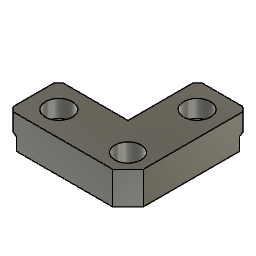
PIU corner bumper v1 (Autodesk Fusion 360 design; units mm, degrees)
Autodesk Fusion 360 part; units mm, degrees
note: some values were not read from the file. Chosen so that the rebuilt part matches the saved one: where a step ends.
sketch "base form" plane through (0, 0, 0) normal (0, 0, 1) x (1, 0, 0)
  line L0 (0, 0) -> (-55, 0)
  line L1 (0, 55) -> (0, 0)
  line L2 (0, 55) -> (-23, 55)
  line L3 (-55, 0) -> (-55, 23)
  line L4 (-55, 23) -> (-23, 23)
  line L5 (-23, 23) -> (-23, 55)
  dimension "d1" = 55
  dimension "d2" = 55
  dimension "d3" = 23
  dimension "d4" = 23
  constraint horizontal L0
  constraint vertical L1
  constraint coincident L0.start L1.end
  constraint perpendicular L1 L2
  constraint perpendicular L0 L3
  constraint horizontal L4
  constraint vertical L5
  measures "d1" distance of L0.start L0.end
  measures "d2" distance of L0.start L1.start
  measures "d3" distance of L1.start L2.end
  measures "d4" distance of L0.end L3.end
extrude "Extrude1" add sketch "base form" along normal blind 15
chamfer "Chamfer1" distance 7 angle 45 1 edges at (0, 0, 7.5)
sketch "frame hole" plane through (0, 0, 15) normal (0, 0, 1) x (-1, 0, 0)
  line L0 (7, 0) -> (0, -7)
  line L1 (0, -7) -> (0, -55)
  line L2 (0, -55) -> (23, -55)
  line L3 (23, -55) -> (23, -23)
  line L4 (23, -23) -> (55, -23)
  line L5 (55, -23) -> (55, 0)
  line L6 (55, 0) -> (7, 0)
  line L7 (3.5, -3.5) -> (5.9749, -5.9749) construction
  line L8 (3.5, -3.5) -> (7, -3.5) construction
  line L9 (5.9749, -5.9749) -> (13.0459, -13.0459) construction
  line L10 (5.9749, -5.9749) -> (15.9749, -5.9749) construction
  circle A0 centre (10.2175, -10.2175) radius 6
  dimension "d8" = 45
  dimension "d9" = 3.5
  dimension "d10" = 45
  dimension "d11" = 10
  dimension "d12" = 12
  constraint horizontal L8
  constraint midpoint L0 L7.start
  constraint horizontal L10
  constraint coincident L7.end A0
  measures "d8" angle of L7 L8
  measures "d9" distance of L7.start L7.end
  measures "d10" angle of L9 L10
  measures "d11" distance of L7.end L9.end
  measures "d12" diameter of A0
sketch "mounting screw holes" plane through (0, 0, 15) normal (0, 0, 1) x (-1, 0, 0)
  line L0 (55, -11.5) -> (49.55, -11.5) construction
  line L1 (55, -23) -> (55, 0) construction
  line L2 (41, 16) -> (41, 11) construction
  line L3 (49.55, -11.5) -> (31, -11.5) construction
  circle A0 centre (43.35, -11.5) radius 6.2
  circle A1 centre (43.35, -11.5) radius 3
  line L4 (3.5, -3.5) -> (10.5711, -10.5711) construction
  line L5 (3.5, -3.5) -> (13.5, -3.5) construction
  line L6 (0, -7) -> (7, 0) construction
  circle A2 centre (11.5, -43.35) radius 6.2
  circle A3 centre (11.5, -43.35) radius 3
  dimension "d13" = 5.45
  dimension "d14" = 5
  dimension "d15" = 12.4
  dimension "d16" = 6
  dimension "d17" = 45
  dimension "d18" = 10
  constraint horizontal L0
  constraint midpoint L0.start L1
  constraint vertical L2
  constraint parallel L0 L3
  constraint coincident L0.end A0
  constraint concentric A0 A1
  constraint horizontal L5
  constraint midpoint L4.start L6
  constraint symmetric A0 L4 A2
  constraint symmetric A1 L4 A3
  measures "d13" distance of L0.start L0.end
  measures "d14" distance of L2.start L2.end
  measures "d15" diameter of A0
  measures "d16" diameter of A1
  measures "d17" angle of L4 L5
  measures "d18" distance of L4.start L4.end
extrude "Extrude2" cut sketch "frame hole" against normal up to surface (15 mm away) contours A0
extrude "Extrude3" cut sketch "mounting screw holes" along normal up to far side of body 1 contours A1 | A3
extrude "Extrude4" cut sketch "mounting screw holes" against normal blind 8
sketch "relief holes" plane through (0, 0, 0) normal (0, 0, -1) x (1, 0, 0)
  circle A0 centre (-43.35, -11.5) radius 3
  circle A1 centre (-11.5, -43.35) radius 3
  circle A2 centre (-10.2175, -10.2175) radius 6
  line L0 (0, -7) -> (-7, 0)
  line L1 (-7, 0) -> (-55, 0)
  line L2 (-55, 0) -> (-55, -23)
  line L3 (-55, -23) -> (-23, -23)
  line L4 (-23, -23) -> (-23, -55)
  line L5 (-23, -55) -> (0, -55)
  line L6 (0, -55) -> (0, -7)
  line L7 (-14, -40.35) -> (-9, -40.35) construction
  line L8 (-11.5, -40.35) -> (-11.5, -33.35) construction
  line L9 (-11.5, -43.35) -> (-11.5, -37.5) construction
  line L10 (-11.5, -33.35) -> (-11.5, -33) construction
  line L11 (-11.5, -33) -> (-11.5, -20) construction
  line L12 (-11.5, -33) -> (-5, -33) construction
  line L13 (-5, -33) -> (-18, -33)
  line L14 (-18, -33) -> (-18, -20)
  line L15 (-18, -20) -> (-5, -20)
  line L16 (-5, -20) -> (-5, -33)
  line L17 (-3.5, -3.5) -> (-10.5711, -10.5711)
  line L18 (-3.5, -3.5) -> (6.5, -3.5) construction
  line L19 (-33, -5) -> (-33, -18)
  line L20 (-33, -18) -> (-20, -18)
  line L21 (-20, -5) -> (-33, -5)
  line L22 (-20, -18) -> (-20, -5)
  dimension "d25" = 5
  dimension "d26" = 7
  dimension "d27" = 13
  dimension "d28" = 6.5
  dimension "d29" = 13
  dimension "d30" = 13
  dimension "d31" = 135
  dimension "d32" = 10
  constraint perpendicular L4 L7
  constraint tangent A1 L7
  constraint midpoint L7 L8.start
  constraint perpendicular L7 L8
  constraint coincident A1.centre L9.start
  constraint vertical L9
  constraint coincident A1 L8.start
  constraint coincident L8.start L9
  constraint parallel L8 L11
  constraint perpendicular L10 L12
  constraint horizontal L13
  constraint vertical L14
  constraint horizontal L15
  constraint vertical L16
  constraint horizontal L18
  constraint midpoint L0 L17.start
  constraint symmetric L12.end L17 L19.start
  constraint symmetric L13.end L17 L19.end
  constraint symmetric L14.end L17 L20.end
  constraint symmetric L15.end L17 L21.start
  measures "d25" distance of L7.start L7.end
  measures "d26" distance of L8.start L8.end
  measures "d27" distance of L10.end L11.end
  measures "d28" distance of L10.end L12.end
  measures "d29" distance of L12.end L13.end
  measures "d30" distance of L12.end L15.end
  measures "d31" angle of L17 L18
  measures "d32" distance of L17.start L17.end
extrude "Extrude5" cut sketch "relief holes" against normal blind 12 contours L13 L14 L15 L16 | L19 L20 L21 L22
chamfer "Chamfer2" distance 2 angle 45 4 edges at (-23, 55, 7.5) (0, 55, 7.5) (-55, 23, 7.5) (-55, 0, 7.5)
sketch "wire routing holes" plane through (0, 0, 0) normal (0, 0, -1) x (1, 0, 0)
  line L0 (-18, -33) -> (-18, -20)
  line L1 (-18, -20) -> (-5, -20)
  line L2 (-5, -20) -> (-5, -33)
  line L3 (-5, -33) -> (-18, -33)
  line L4 (-33, -5) -> (-20, -5)
  line L5 (-20, -5) -> (-20, -18)
  line L6 (-20, -18) -> (-33, -18)
  line L7 (-33, -18) -> (-33, -5)
  circle A0 centre (-43.35, -11.5) radius 3
  circle A1 centre (-11.5, -43.35) radius 3
  circle A2 centre (-10.2175, -10.2175) radius 6
  line L8 (-53, 0) -> (-55, -2)
  line L9 (-55, -2) -> (-55, -21)
  line L10 (-55, -21) -> (-53, -23)
  line L11 (-53, -23) -> (-23, -23)
  line L12 (-23, -23) -> (-23, -53)
  line L13 (-23, -53) -> (-21, -55)
  line L14 (-21, -55) -> (-2, -55)
  line L15 (-2, -55) -> (0, -53)
  line L16 (0, -53) -> (0, -7)
  line L17 (0, -7) -> (-7, 0)
  line L18 (-7, 0) -> (-53, 0)
  line L19 (-55, -23) -> (-51.5, -23) construction
  line L20 (-51.5, -23) -> (-55, -23)
  line L21 (-55, -23) -> (-55, 0)
  line L22 (-55, 0) -> (-51.5, 0)
  line L23 (-51.5, 0) -> (-51.5, -23)
  line L24 (-3.5, -3.5) -> (-10.5711, -10.5711)
  line L25 (-23, -55) -> (0, -55)
  line L26 (0, -55) -> (0, -51.5)
  line L27 (-23, -51.5) -> (-23, -55)
  line L28 (0, -51.5) -> (-23, -51.5)
  dimension "d36" = 3.5
  constraint perpendicular L9 L19
  constraint horizontal L20
  constraint vertical L21
  constraint horizontal L22
  constraint vertical L23
  constraint symmetric L19.end L24 L27.start
  constraint symmetric L19.start L24 L25.start
  constraint symmetric L21.end L24 L25.end
  constraint symmetric L22.end L24 L26.end
  measures "d36" distance of L19.start L19.end
extrude "Extrude6" cut sketch "wire routing holes" against normal blind 3.5 contours L8 L9 L10 L11 L18 L20 L21 L22 L23 | L12 L13 L14 L15 L16 L25 L26 L27 L28
chamfer "Chamfer3" distance 3.499 angle 45 6 edges at (-11.5, 55, 3.5) (-55, 11.5, 3.5) (-54, 22, 3.5) (-54, 1, 3.5) (-22, 54, 3.5) (-1, 54, 3.5)
equation "d28 = ( 13 / 2 ) * 1 mm"
named bodies: "Corner bumper"
